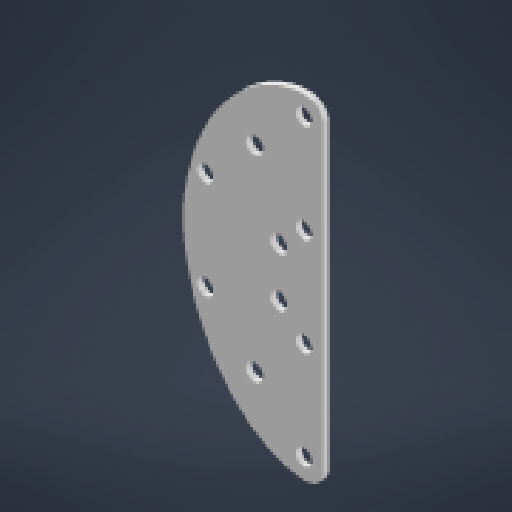
# Autodesk Inventor part: shaft-retainer-v2
Saved by Autodesk Inventor 2024 (Build 280153000, 153)
## iProperties
Created: 2023-04-20
Part Number: shaft-retainer-v2
Material: Generic
Document SubType Name: Modeling
Designer: liamt
Density: 1 g/cm^3
Appearance: Default
Author: liamt
Autodesk Inventor part; units mm, degrees
ref_plane "YZ Plane" through (0, 0, 0) normal (1, 0, 0) x (0, 1, 0)
ref_plane "XZ Plane" through (0, 0, 0) normal (0, 1, 0) x (-1, 0, 0)
ref_plane "XY Plane" through (0, 0, 0) normal (0, 0, 1) x (1, 0, 0)
sketch "Sketch1" plane through (0, 0, 0) normal (0, 0, 1) x (1, 0, 0)
  line L0 (11.43, -25.4) -> (11.43, -76.2)
  circle A0 centre (6.35, -38.1) radius 2.0955
  circle A1 centre (6.35, -63.5) radius 2.0955
  line L1 (11.43, -76.2) -> (11.43, -88.9)
  line L2 (11.43, -25.4) -> (11.43, -12.7)
  circle A2 centre (6.35, -12.7) radius 2.0955
  circle A3 centre (6.35, -88.9) radius 2.0955
  line L3 (6.35, -38.1) -> (6.35, -63.5) construction
  line L4 (6.35, -50.8) -> (8.4455, -50.8) construction
  line L5 (6.35, -7.62) -> (-1.2208, -7.62) construction
  line L6 (-1.2208, -7.62) -> (-21.1455, -14.7955) construction
  line L7 (-21.1455, -14.7955) -> (-24.8856, -42.1223) construction
  line L8 (-24.8856, -42.1223) -> (-24.8856, -50.8) construction
  spline S0 degree 4 poles (6.35, -7.62) (-1.2208, -7.62) (-21.1455, -14.7955) (-24.8856, -42.1223) (-24.8856, -50.8) knots 1 1 1 1 1 2 2 2 2 2
  line L9 (6.35, -93.98) -> (-1.2208, -93.98) construction
  line L10 (-1.2208, -93.98) -> (-21.1455, -86.8045) construction
  line L11 (-21.1455, -86.8045) -> (-24.8856, -59.4777) construction
  line L12 (-24.8856, -59.4777) -> (-24.8856, -50.8) construction
  spline S1 degree 4 poles (6.35, -93.98) (-1.2208, -93.98) (-21.1455, -86.8045) (-24.8856, -59.4777) (-24.8856, -50.8) knots 1 1 1 1 1 2 2 2 2 2
  spline S2 degree 4 poles (11.43, -12.7) (11.43, -11.6705) (11.43, -9.6114) (9.4386, -7.8854) (7.3795, -7.62) (6.35, -7.62) knots 0 0 0 0 0 0.5 1 1 1 1 1
  spline S3 degree 4 poles (11.43, -88.9) (11.43, -89.9295) (11.43, -91.9886) (9.4386, -93.7146) (7.3795, -93.98) (6.35, -93.98) knots 0 0 0 0 0 0.5 1 1 1 1 1
  circle A4 centre (-6.35, -25.4) radius 2.1844 projected
  circle A5 centre (-6.35, -76.2) radius 2.1844 projected
  circle A6 centre (0, -44.45) radius 2.1844 projected
  circle A7 centre (0, -57.15) radius 2.1844 projected
  line L13 (-12.7, -30.6578) -> (-12.7, 30.8102) projected
  circle A8 centre (-19.05, -38.1) radius 2.0955
  circle A9 centre (-19.05, -63.5) radius 2.0955
  point P0 (0, 0)
  dimension "d2" = 4.191
  dimension "d3" = 4.191
  dimension "d4" = 12.7
  dimension "d5" = 4.191
  dimension "d6" = 4.191
  dimension "d9" = 4.191
  dimension "d10" = 6.35
  dimension "d12" = 0
  dimension "d13" = 4.191
  dimension "d14" = 0
  dimension "d15" = 0
  constraints: 10 end point, 6 centre point, 5 vertical, 4 symmetric about line, 2 horizontal, 1 midpoint, 16 other
  measures "d2" diameter of A1
  measures "d3" diameter of A0
  measures "d4" distance of L0.start L2.end
  measures "d5" diameter of A2
  measures "d6" diameter of A3
  measures "d9" diameter of A8
  measures "d10" distance from line of L13 A8.centre
  measures "d12" vertical distance of L3.start A8.centre
  measures "d13" diameter of A9
  measures "d14" vertical distance of L3.end A9.centre
  measures "d15" horizontal distance of A8.centre A9.centre
extrude "Extrusion2" add sketch "Sketch1" along normal blind 1.524
body "Solid2"
